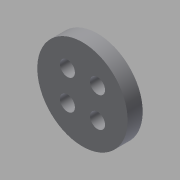
# Autodesk Inventor part: ShoulderBracketXZPlate
Saved by Autodesk Inventor 2017 (Build 210142000, 142)
## iProperties
Created: 2017-05-07
Part Number: ShoulderBracketXZPlate
Material: Generic
Document SubType Name: Modeling
Designer: zallen
Density: 1 g/cm^3
Appearance: Default
Author: zallen
Autodesk Inventor part; units mm, degrees
ref_plane "YZ Plane" through (0, 0, 0) normal (1, 0, 0) x (0, 1, 0)
ref_plane "XZ Plane" through (0, 0, 0) normal (0, 1, 0) x (-1, 0, 0)
ref_plane "XY Plane" through (0, 0, 0) normal (0, 0, 1) x (1, 0, 0)
sketch "Sketch1" plane through (0, 0, 0) normal (0, 0, 1) x (1, 0, 0)
  circle A0 centre (0, 0) radius 19.05
  circle A1 centre (6.35, 6.35) radius 3.175
  circle A2 centre (-6.35, 6.35) radius 3.175
  circle A3 centre (-6.35, -6.35) radius 3.175
  circle A4 centre (6.35, -6.35) radius 3.175
  line L0 (0, 0) -> (0, 38.1233) construction
  line L1 (0, 0) -> (30.2858, 0) construction
  dimension "d0" = 38.1
  dimension "d1" = 6.35
  dimension "d4" = 360
  dimension "d6" = 6.35
  dimension "d7" = 6.35
  constraints: 5 centre point, 4 end point, 1 coincident, 1 horizontal, 1 vertical, 9 other
  measures "d0" diameter of A0
  measures "d1" diameter of A1
  measures "d6" distance from line of L0 A1.centre
  measures "d7" distance from line of L1 A1.centre
extrude "Extrusion1" add sketch "Sketch1" along normal blind 6.35
body "Solid1"
